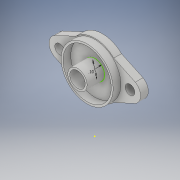
# Autodesk Inventor part: Ball Baering
Saved by Autodesk Inventor 2019 (Build 230136000, 136)
## iProperties
Created: 2021-06-23
Part Number: Ball Baering
Material: Generic
Document SubType Name: Modeling
Designer: 91742
Density: 1 g/cm^3
Appearance: Default
Author: 91742
Autodesk Inventor part; units mm, degrees
ref_plane "YZ Plane" through (0, 0, 0) normal (1, 0, 0) x (0, 1, 0)
ref_plane "XZ Plane" through (0, 0, 0) normal (0, 1, 0) x (-1, 0, 0)
ref_plane "XY Plane" through (0, 0, 0) normal (0, 0, 1) x (1, 0, 0)
sketch "Sketch1" plane through (0, 0, 0) normal (0, 0, 1) x (1, 0, 0)
  circle A0 centre (-18.25, 30) radius 2.5
  circle A1 centre (0, 30) radius 13.5
  line L0 (-18.25, 30) -> (-12.75, 30) construction
  line L1 (-18.25, 30) -> (-12.75, 30) construction
  arc A2 (-21, 34.7631) -> (-21, 25.2369) centre (-18.25, 30) ccw
  line L2 (-21, 34.7631) -> (-1.6262, 34.7631) construction
  line L3 (-21, 25.2369) -> (-9.8237, 20.0252)
  line L4 (-21, 25.2369) -> (-7.9961, 25.2369) construction
  line L5 (-21, 34.7631) -> (-9.8237, 39.9748)
  circle A3 centre (18.25, 30) radius 2.5
  line L6 (18.25, 30) -> (12.75, 30) construction
  line L7 (18.25, 30) -> (12.75, 30) construction
  arc A4 (21, 25.2369) -> (21, 34.7631) centre (18.25, 30) ccw
  line L8 (21, 34.7631) -> (1.6262, 34.7631) construction
  line L9 (21, 25.2369) -> (9.8237, 20.0252)
  line L10 (21, 25.2369) -> (7.9961, 25.2369) construction
  line L11 (21, 34.7631) -> (9.8237, 39.9748)
  arc A5 (-9.8237, 20.0252) -> (9.8237, 20.0252) centre (0, 30) ccw
  arc A6 (9.8237, 39.9748) -> (-9.8237, 39.9748) centre (0, 30) ccw
  point P0 (0, 0)
  dimension "d0" = 5
  dimension "d8" = 27
  dimension "d13" = 25
  constraints: 24 end point, 8 point on circle, 7 centre point, 5 coincident, 4 horizontal
  measures "d0" diameter of A0
  measures "d8" diameter of A1
  measures "d13" angle of L3 L4
extrude "Extrusion1" add sketch "Sketch1" along normal blind 4
sketch "Sketch2" plane through (0, 0, 4) normal (0, 0, 1) x (1, 0, 0)
  circle A0 centre (0, 30) radius 13.5
  point P0 (0, 0)
  dimension "d16" = 27
  constraints: 1 centre point
  measures "d16" diameter of A0
extrude "Extrusion2" add sketch "Sketch2" against normal blind 4
sketch "Sketch3" plane through (0, 0, 4) normal (0, 0, 1) x (1, 0, 0)
  circle A0 centre (0, 30) radius 13.5
  circle A1 centre (0, 30) radius 12.5
  point P0 (0, 0)
  dimension "d19" = 27
  dimension "d20" = 25
  constraints: 2 centre point, 2 coincident
  measures "d19" diameter of A0
  measures "d20" diameter of A1
extrude "Extrusion3" add sketch "Sketch3" along normal blind 4
sketch "Sketch4" plane through (0, 30, 4) normal (0, 0, 1) x (1, 0, 0)
  circle A0 centre (0, 0) radius 5
  circle A1 centre (0, 0) radius 4
  point P0 (0, -30)
  dimension "d23" = 10
  dimension "d24" = 8
  constraints: 2 centre point, 1 coincident
  measures "d23" diameter of A0
  measures "d24" diameter of A1
extrude "Extrusion4" add sketch "Sketch4" along normal blind 9
body "Solid1"
